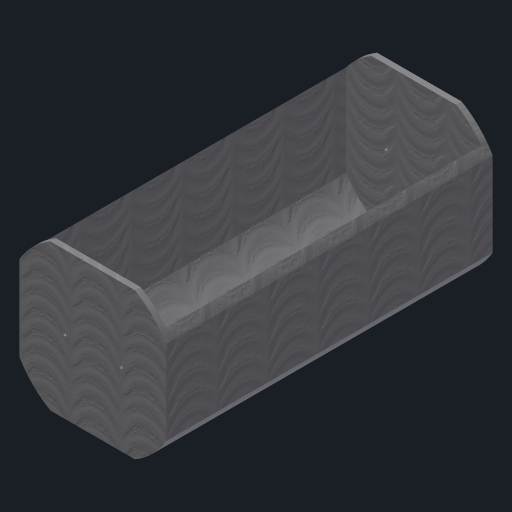
# Autodesk Inventor part: CAJA_V2
Saved by Autodesk Inventor 2024.3 (Build 283343000, 343)
## iProperties
Created: 2024-07-12
Part Number: CAJA_V2
Material: Steel, Mild, Welded
Document SubType Name: Modeling
Designer: Niler
Density: 7.85 g/cm^3
Appearance: Weld - Steel Mild
Author: Niler
Autodesk Inventor part; units mm, degrees
ref_plane "YZ Plane" through (0, 0, 0) normal (1, 0, 0) x (0, 1, 0)
ref_plane "XZ Plane" through (0, 0, 0) normal (0, 1, 0) x (-1, 0, 0)
ref_plane "XY Plane" through (0, 0, 0) normal (0, 0, 1) x (1, 0, 0)
sketch "Sketch1" plane through (0, 0, 0) normal (0, 1, 0) x (-1, 0, 0)
  line L0 (-65, 145) -> (65, 145)
  line L1 (65, 145) -> (65, -145)
  line L2 (65, -145) -> (-65, -145)
  line L3 (-65, -145) -> (-65, 145)
  line L4 (-65, 145) -> (65, -145) construction
  line L5 (65, 145) -> (-65, -145) construction
  point P0 (0, 0)
  dimension "d0" = 130
  dimension "d1" = 290
  constraints: 12 end point, 2 midpoint, 2 parallel, 1 horizontal, 1 perpendicular
  measures "d0" distance of L1.end L2.end
  measures "d1" distance of L0.end L1.end
extrude "Extrusion1" add sketch "Sketch1" along normal blind 130
sketch "Sketch2" plane through (-65, 0, 145) normal (0, 0, 1) x (1, 0, 0)
  line L0 (0, 0) -> (130, 0) projected
  line L1 (130, 0) -> (130, 130) projected
  line L2 (0, 130) -> (130, 130) projected
  line L3 (0, 0) -> (0, 130) projected
  circle A0 centre (65, 65) radius 75
  point P0 (65, 0)
  point P1 (130, 65)
  point P2 (65, 130)
  point P3 (27.5834, 0)
  point P4 (0, 27.5834)
  point P5 (130, 27.5834)
  point P6 (102.4166, 0)
  point P7 (0, 102.4166)
  point P8 (27.5834, 130)
  point P9 (102.4166, 130)
  point P10 (130, 102.4166)
  dimension "d4" = 150
  constraints: 2 midpoint, 1 centre point, 1 horizontal alignment, 1 vertical alignment
  measures "d4" diameter of A0
extrude "Extrusion2" cut sketch "Sketch2" against normal through all contours L3 A0 L0 | A0 L1 L0 | L3 L2 A0 | A0 L2 L1
sketch "Sketch3" plane through (0, 130, 0) normal (0, 1, 0) x (1, 0, 0)
  line L0 (-37.4166, 145) -> (-37.4166, -145) projected
  line L1 (-37.4166, -145) -> (37.4166, -145) projected
  line L2 (37.4166, -145) -> (37.4166, 145) projected
  line L3 (37.4166, 145) -> (-37.4166, 145) projected
  line L4 (37.4166, 145) -> (65, 145) projected
  line L5 (37.4166, -145) -> (37.4166, 145) projected
  line L6 (65, -145) -> (37.4166, -145) projected
  line L7 (65, 145) -> (65, -145) projected
  line L8 (-65, 145) -> (-37.4166, 145) projected
  line L9 (-65, -145) -> (-65, 145) projected
  line L10 (-37.4166, -145) -> (-65, -145) projected
  line L11 (-37.4166, 145) -> (-37.4166, -145) projected
  line L12 (-60, -140) -> (60, -140)
  line L13 (60, -140) -> (60, 140)
  line L14 (60, 140) -> (-60, 140)
  line L15 (-60, 140) -> (-60, -140)
  line L16 (-60, -140) -> (60, 140) construction
  line L17 (60, -140) -> (-60, 140) construction
  point P0 (0, 0)
  dimension "d7" = 5
  dimension "d8" = 5
  constraints: 12 end point, 2 midpoint, 2 parallel, 1 horizontal, 1 perpendicular
  measures "d7" distance between parallel lines of L7 L13
  measures "d8" distance between parallel lines of L3 L14
extrude "Extrusion3" cut sketch "Sketch3" against normal through all contours L14 L2 L12 L0 | L0 L12 L15 L14 | L14 L13 L12 L2
sketch "Sketch4" plane through (-37.4166, 0, 145) normal (0, 0, 1) x (1, 0, 0)
  arc A0 (74.8331, 0) -> (102.4166, 27.5834) centre (37.4166, 65) ccw projected
  line L0 (102.4166, 27.5834) -> (102.4166, 102.4166) projected
  arc A1 (102.4166, 102.4166) -> (74.8331, 130) centre (37.4166, 65) ccw projected
  line L1 (0, 130) -> (74.8331, 130) projected
  arc A2 (0, 130) -> (-27.5834, 102.4166) centre (37.4166, 65) ccw projected
  line L2 (-27.5834, 27.5834) -> (-27.5834, 102.4166) projected
  arc A3 (-27.5834, 27.5834) -> (0, 0) centre (37.4166, 65) ccw projected
  line L3 (0, 0) -> (74.8331, 0) projected
  arc A4 (-22.5834, 28.9445) -> (1.3611, 5) centre (37.4166, 65) ccw
  line L4 (-22.5834, 28.9445) -> (-22.5834, 101.0555)
  arc A5 (1.3611, 125) -> (-22.5834, 101.0555) centre (37.4166, 65) ccw
  line L5 (1.3611, 125) -> (73.4721, 125)
  arc A6 (97.4166, 101.0555) -> (73.4721, 125) centre (37.4166, 65) ccw
  line L6 (97.4166, 101.0555) -> (97.4166, 28.9445)
  arc A7 (73.4721, 5) -> (97.4166, 28.9445) centre (37.4166, 65) ccw
  line L7 (73.4721, 5) -> (1.3611, 5)
  line L8 (-27.5834, 27.5834) -> (-22.5834, 28.9445)
  line L9 (97.4166, 28.9445) -> (102.4166, 27.5834)
  point P0 (37.4166, 0)
  dimension "d11" = 5
  constraints: 12 end point, 8 point on circle, 4 centre point, 7 other
  measures "d11" radial gap between concentric circles of A3 A4
extrude "Extrusion4" add sketch "Sketch4" against normal up to surface (290 mm away) contours L3 A3 L8 A4 L7 A7 L9 A0
sketch "Sketch5" plane through (-37.4166, 0, 145) normal (0, 0, 1) x (1, 0, 0)
  line L0 (102.4166, 27.5834) -> (102.4166, 102.4166) projected
  arc A0 (102.4166, 102.4166) -> (74.8331, 130) centre (37.4166, 65) ccw projected
  line L1 (0, 130) -> (74.8331, 130) projected
  arc A1 (0, 130) -> (-27.5834, 102.4166) centre (37.4166, 65) ccw projected
  line L2 (-27.5834, 27.5834) -> (-27.5834, 102.4166) projected
  arc A2 (-27.5834, 27.5834) -> (0, 0) centre (37.4166, 65) ccw projected
  line L3 (0, 0) -> (74.8331, 0) projected
  arc A3 (74.8331, 0) -> (102.4166, 27.5834) centre (37.4166, 65) ccw projected
  line L4 (12.4166, 65) -> (62.4166, 65) construction
  circle A4 centre (62.4166, 65) radius 1.65
  circle A5 centre (12.4166, 65) radius 1.65
  point P0 (37.4166, 0)
  dimension "d14" = 3.3
  dimension "d15" = 3.3
  dimension "d16" = 50
  constraints: 3 coincident, 2 centre point, 2 end point, 1 horizontal, 1 midpoint
  measures "d14" diameter of A4
  measures "d15" diameter of A5
  measures "d16" distance of L4.start L4.end
extrude "Extrusion5" cut sketch "Sketch5" against normal through all contours A4 | A5
body "Solid1"
